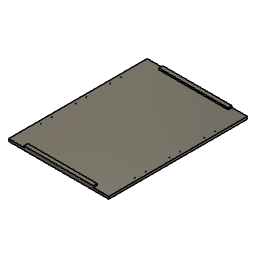
Chasis Sumo v1 (Autodesk Fusion 360 design; units mm, degrees)
Autodesk Fusion 360 part; units mm, degrees
sketch "Esquisse1" plane through (0, 0, 0) normal (0, 1, 0) x (1, 0, 0)
  line L0 (0, 0) -> (130, 0)
  line L1 (130, 0) -> (130, -180)
  line L2 (130, -180) -> (0, -180)
  line L3 (0, -180) -> (0, 0)
  line L4 (130, -97.0172) -> (126, -97.0172)
  circle A0 centre (126, -97.0172) radius 0.5
  circle A1 centre (126, -82.9828) radius 0.5
  line L5 (130, -82.9828) -> (126, -82.9828)
  line L6 (130, -52.0186) -> (126, -52.0186)
  circle A2 centre (126, -52.0186) radius 0.5
  circle A3 centre (126, -37.9814) radius 0.5
  line L7 (130, -37.9814) -> (126, -37.9814)
  line L8 (130, -142.0186) -> (126, -142.0186)
  line L9 (130, -127.9814) -> (126, -127.9814)
  circle A4 centre (126, -142.0186) radius 0.5
  circle A5 centre (126, -127.9814) radius 0.5
  line L10 (0, -37.9814) -> (4, -37.9814)
  circle A6 centre (4, -37.9814) radius 0.5
  line L11 (0, -52.0186) -> (4, -52.0186)
  line L12 (0, -82.9828) -> (4, -82.9828)
  circle A7 centre (4, -82.9828) radius 0.5
  line L13 (0, -97.0172) -> (4, -97.0172)
  circle A8 centre (4, -127.9814) radius 0.5
  line L14 (0, -127.9814) -> (4, -127.9814)
  line L15 (0, -142.0186) -> (4, -142.0186)
  circle A9 centre (4, -142.0186) radius 0.5
  line L16 (65, 0) -> (65, -180)
  circle A10 centre (4, -52.0186) radius 0.5
  circle A11 centre (4, -97.0172) radius 0.5
  point P0 (4, -52.0186)
  point P1 (4, -97.0172)
  dimension "d1" = 130
  dimension "d2" = 180
  dimension "d5" = 4
  dimension "d6" = 1
  dimension "d8" = 4
  dimension "d9" = 1
  constraint horizontal L0
  constraint vertical L1
  constraint horizontal L2
  constraint vertical L3
  constraint coincident L0.start L3.end
  constraint coincident L1 L4.start
  constraint perpendicular L1 L4
  constraint coincident L4.end A0.centre
  constraint coincident L1 L6.start
  constraint perpendicular L1 L6
  constraint coincident L6.end A2.centre
  constraint midpoint L0 L16.start
  constraint midpoint L2 L16.end
  constraint symmetric A0 L16 A11
  constraint symmetric A2 L16 A10
  measures "d1" distance of L0.start L0.end
  measures "d2" distance of L0.start L2.end
  measures "d5" distance of L4.start L4.end
  measures "d6" diameter of A0
  measures "d8" distance of L6.start L6.end
  measures "d9" diameter of A2
extrude "Extrusion1" add sketch "Esquisse1" along normal blind 3
sketch "Esquisse2" plane through (0, 3, 0) normal (0, 1, 0) x (-1, 0, 0)
  circle A0 centre (-126, 127.9814) radius 0.5
  circle A1 centre (-126, 97.0172) radius 0.5
  circle A2 centre (-126, 82.9828) radius 0.5
  circle A3 centre (-126, 52.0186) radius 0.5
  circle A4 centre (-126, 37.9814) radius 0.5
  circle A5 centre (-4, 37.9814) radius 0.5
  circle A6 centre (-4, 97.0172) radius 0.5
  circle A7 centre (-4, 82.9828) radius 0.5
  circle A8 centre (-4, 52.0186) radius 0.5
  circle A9 centre (-4, 127.9814) radius 0.5
  circle A10 centre (-126, 142.0186) radius 0.5
  circle A11 centre (-4, 142.0186) radius 0.5
  line L0 (0, 180) -> (-130, 180)
  line L1 (-130, 180) -> (-130, 0)
  line L2 (-130, 0) -> (0, 0)
  line L3 (0, 0) -> (0, 180)
  line L4 (-20, 0) -> (-110, 0)
  line L5 (-110, 0) -> (-110, 5)
  line L6 (-110, 5) -> (-20, 5)
  line L7 (-20, 5) -> (-20, 0)
  line L8 (-110, 175) -> (-20, 175)
  line L9 (-110, 180) -> (-110, 175)
  line L10 (-20, 180) -> (-110, 180)
  line L11 (-20, 175) -> (-20, 180)
  constraint horizontal L4
  constraint vertical L5
  constraint horizontal L6
  constraint vertical L7
  constraint coincident L2 L4.start
extrude "Extrusion2" add sketch "Esquisse2" along normal blind 2 contours L0 L8 L9 L10 L11 | L2 L4 L5 L6 L7
